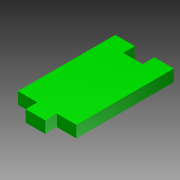
# Autodesk Inventor part: servo_holder3
Saved by Autodesk Inventor 2012 (Build 160160000, 160)
## iProperties
Created: 2013-10-03
Part Number: servo_holder3
Material: Default
Document SubType Name: Modeling
Designer: Nick
Density: 1 g/cm^3
Author: Nick
Autodesk Inventor part; units mm, degrees
ref_plane "YZ Plane" through (0, 0, 0) normal (1, 0, 0) x (0, 1, 0)
ref_plane "XZ Plane" through (0, 0, 0) normal (0, 1, 0) x (-1, 0, 0)
ref_plane "XY Plane" through (0, 0, 0) normal (0, 0, 1) x (1, 0, 0)
sketch "Sketch1" plane through (0, 0, 0) normal (0, 0, 1) x (1, 0, 0)
  line L0 (15, 0) -> (15, 25)
  line L1 (0, 25) -> (0, 0)
  line L2 (10, 0) -> (10, -3)
  line L3 (10, -3) -> (5, -3)
  line L4 (5, -3) -> (5, 0)
  line L5 (10, 25) -> (10, 22)
  line L6 (10, 22) -> (5, 22)
  line L7 (5, 22) -> (5, 25)
  line L8 (15, 25) -> (10, 25)
  line L9 (5, 25) -> (0, 25)
  line L10 (0, 0) -> (5, 0)
  line L11 (10, 0) -> (15, 0)
  dimension "d0" = 15
  dimension "d1" = 25
  dimension "d2" = 5
  dimension "d3" = 3
  dimension "d4" = 5
  dimension "d6" = 5
  dimension "d7" = 3
  constraints: 24 end point, 7 parallel, 3 horizontal, 2 horizontal alignment, 2 perpendicular, 2 vertical alignment
  measures "d0" distance of L1.start L0.end
  measures "d1" distance of L0.end L0.start
  measures "d2" distance of L2.end L3.end
  measures "d3" distance of L2.start L2.end
  measures "d4" distance of L6.end L5.end
  measures "d6" distance between parallel lines of L7 L1
  measures "d7" distance of L5.start L5.end
extrude "Extrusion1" add sketch "Sketch1" along normal blind 3
equation "\"d6\" = 0.5 * d0 - 0.5 * d4"
body "Solid1"
